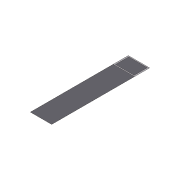
# Autodesk Inventor part: Frame_CrossbarAngleSupport_FrontRear_Horizontal
Saved by Autodesk Inventor 2012 (Build 160160000, 160)
## iProperties
Created: 2012-01-13
Part Number: Frame_CrossbarAngleSupport_FrontRear_Horizontal
Material: Aluminum-6061
Document SubType Name: Modeling
Designer: JesseK
Mass: 345.421 g
Surface Area: 218.975 cm^2
Volume: 127.461 cm^3
Density: 2.71 g/cm^3
Author: JesseK
Autodesk Inventor part; units mm, degrees
ref_plane "YZ Plane" through (0, 0, 0) normal (1, 0, 0) x (0, 1, 0)
ref_plane "XZ Plane" through (0, 0, 0) normal (0, 1, 0) x (-1, 0, 0)
ref_plane "XY Plane" through (0, 0, 0) normal (0, 0, 1) x (1, 0, 0)
sketch "Sketch1" plane through (0, 0, 0) normal (0, 0, 1) x (1, 0, 0)
  line L0 (0, 0) -> (35.921, 0)
  line L1 (35.921, 0) -> (175.621, 139.7)
  line L2 (175.621, 139.7) -> (139.7, 139.7)
  line L3 (139.7, 139.7) -> (0, 0)
  dimension "d1" = 25.4
  dimension "d2" = 45
  dimension "d3" = 139.7
  constraints: 8 end point, 2 horizontal, 1 parallel
  measures "d1" distance between parallel lines of L1 L3
  measures "d2" angle of L2 L1
  measures "d3" distance between parallel lines of L0 L2
extrude "Extrusion1" add sketch "Sketch1" along normal blind 25.4
shell "Shell1" thickness 1.5875 removed faces 2 at (163.6473, 139.7, 16.9333) at (11.9737, 0, 8.4667)
body "Solid1"
